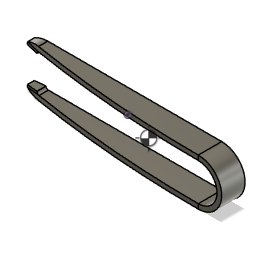
Tweezers v2 (Autodesk Fusion 360 design; units mm, degrees)
Autodesk Fusion 360 part; units mm, degrees
sketch "Sketch1" plane through (0, 0, 0) normal (0, 0, 1) x (1, 0, 0)
sketch "Sketch2" plane through (0, 0, 0) normal (0, 0, 1) x (1, 0, 0)
sketch "Sketch3" plane through (0, 0, 0) normal (0, 0, 1) x (1, 0, 0)
  line L0 (-40, 10) -> (40, 10)
  line L1 (40, -10) -> (-40, -10)
  line L2 (-40, 10) -> (40, -10) construction
  line L3 (40, 10) -> (-40, -10) construction
  arc A0 (40, -10) -> (40, 10) centre (40, 0) ccw
  arc A1 (40, -8) -> (40, 8) centre (40, 0) ccw
  line L4 (-35, 8) -> (40, 8)
  line L5 (40, -8) -> (-35, -8)
  line L6 (-40, -10) -> (-40, -8.4374)
  line L7 (-40, 8.4374) -> (-40, 10)
  line L8 (-35, 8) -> (-40, 8.4374)
  line L9 (-35, -8) -> (-40, -8.4374)
  dimension "d4" = 5
  dimension "d6" = 5
  constraint horizontal L0
  constraint parallel L0 L1
  constraint coincident L2 origin
  constraint coincident L3 origin
  constraint concentric A0 A1
  constraint parallel L0 L4
  constraint parallel L1 L5
  constraint collinear L6 L7
  measures "d4" angle of L4 L8
  measures "d6" angle of L5 L9
extrude "Extrude1" add sketch "Sketch3" along normal blind 10
sketch "Sketch4" plane through (0, -10, 0) normal (0, -1, 0) x (1, 0, 0)
  line L0 (-40, 0) -> (40, 0)
  line L1 (40, 0) -> (40, 10)
  line L2 (40, 10) -> (-40, 10)
  line L3 (-40, 10) -> (-40, 0)
  arc A0 (40, 10) -> (-40, 3) centre (40, -450.6429) ccw
  point P0 (40, 10)
  point P1 (40, 0)
  point P2 (-40, 0)
  point P3 (-40, 10)
  point P4 (-40, 3)
  dimension "d9" = 3
  constraint coincident L3 P4
  constraint tangent L2 A0
  constraint coincident P4 A0.end
  constraint coincident P0 L1.end
  measures "d9" distance of P2 P4
extrude "Extrude2" cut sketch "Sketch4" against normal blind 35 contours L2 L3 A0
extrude "Extrude3" add 1 faces at (-37.5004, 8.2188, 1.1445) along direction (-0.087156, -0.996195, 0) blind 1
extrude "Extrude4" add 1 faces at (-37.5004, -8.2188, 1.1445) along direction (-0.087156, 0.996195, 0) blind 1
fillet "Fillet1" radius 1 2 edges at (-35, 8, 1.9267) (-35, -8, 1.9267)
fillet "Fillet2" radius 11 2 edges at (-40, -10, 1.5) (-40, 10, 1.5)
